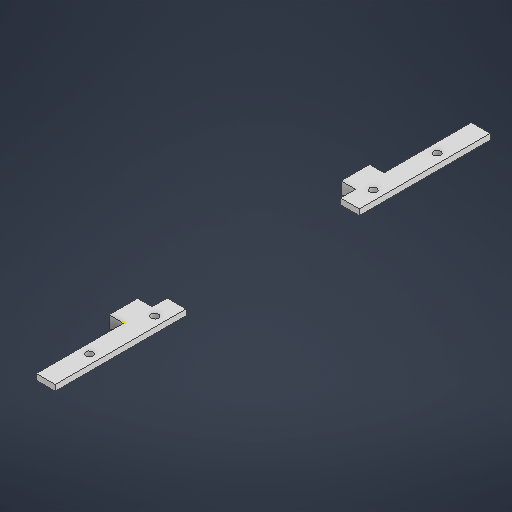
# Autodesk Inventor part: mocowanie do pługu
Saved by Autodesk Inventor 2026.2 (Build 302298010, 298A)
## iProperties
Created: 2026-05-09
Part Number: mocowanie do pługu
Material: Ogólny
Document SubType Name: Modeling
Designer: karol
Density: 1 g/cm^3
Appearance: Domyślna
Author: karol
Autodesk Inventor part; units mm, degrees
ref_plane "YZ Plane" through (0, 0, 0) normal (1, 0, 0) x (0, 1, 0)
ref_plane "XZ Plane" through (0, 0, 0) normal (0, 1, 0) x (-1, 0, 0)
ref_plane "XY Plane" through (0, 0, 0) normal (0, 0, 1) x (1, 0, 0)
sketch "Sketch21" plane through (0, 0, 0) normal (0, 1, 0) x (-1, 0, 0)
  line L0 (0, 0) -> (5, 0)
  line L1 (5, 0) -> (5, -9.8)
  line L2 (5, -9.8) -> (0, -9.8)
  line L3 (0, -9.8) -> (0, 0)
  line L4 (0, -79.8) -> (5, -79.8)
  line L5 (5, -79.8) -> (5, -89.6)
  line L6 (5, -89.6) -> (0, -89.6)
  line L7 (0, -89.6) -> (0, -79.8)
  dimension "d144" = 5
  dimension "d145" = 9.8
  dimension "d146" = 5
  dimension "d147" = 9.8
  dimension "d148" = 70
  constraints: 16 end point, 4 parallel, 2 horizontal, 2 perpendicular
  measures "d144" distance of L1.end L2.end
  measures "d145" distance of L0.end L1.end
  measures "d146" distance of L5.end L6.end
  measures "d147" distance of L4.end L5.end
  measures "d148" distance between parallel lines of L2 L4
extrude "Extrusion19" add sketch "Sketch21" along normal blind 4
sketch "Sketch22" plane through (0, 0, 0) normal (1, 0, 0) x (0, 0, -1)
  line L0 (9.8, 4) -> (0, 4) projected
  line L1 (9.8, 0) -> (9.8, 4) projected
  line L2 (0, 4) -> (9.8, 4)
  line L3 (9.8, 4) -> (9.8, 2)
  line L4 (9.8, 2) -> (0, 2)
  line L5 (0, 2) -> (0, 4)
  line L6 (9.8, 4) -> (15, 4)
  line L7 (15, 4) -> (15, 2)
  line L8 (15, 2) -> (9.8, 2)
  line L9 (9.8, 2) -> (9.8, 4)
  line L10 (0, 4) -> (-30, 4)
  line L11 (-30, 4) -> (-30, 2)
  line L12 (-30, 2) -> (0, 2)
  line L13 (0, 2) -> (0, 4)
  line L14 (89.6, 0) -> (89.6, 4) projected
  line L15 (79.8, 4) -> (89.6, 4)
  line L16 (89.6, 4) -> (89.6, 2)
  line L17 (89.6, 2) -> (79.8, 2)
  line L18 (79.8, 2) -> (79.8, 4)
  line L19 (79.8, 2) -> (74.6, 2)
  line L20 (74.6, 2) -> (74.6, 4)
  line L21 (74.6, 4) -> (79.8, 4)
  line L22 (79.8, 4) -> (79.8, 2)
  line L23 (89.6, 4) -> (119.6, 4)
  line L24 (119.6, 4) -> (119.6, 2)
  line L25 (119.6, 2) -> (89.6, 2)
  line L26 (89.6, 2) -> (89.6, 4)
  point P0 (0, 0)
  point P1 (9.8, 3)
  point P2 (0, 3)
  dimension "d151" = 9.8
  dimension "d152" = 5.2
  dimension "d153" = 30
  dimension "d154" = 5.2
  dimension "d155" = 30
  constraints: 48 end point, 12 parallel, 6 horizontal, 6 perpendicular, 4 midpoint, 2 point on line
  measures "d151" distance of point (9.8, 3) point (0, 3)
  measures "d152" distance of L7.end L8.end
  measures "d153" distance of L12.end L11.end
  measures "d154" distance of L20.end L21.end
  measures "d155" distance of L24.end L25.end
extrude "Extrusion20" add sketch "Sketch22" along normal blind 6.5
sketch "Sketch23" plane through (0, 4, 0) normal (0, 1, 0) x (1, 0, 0)
  point P0 (0, 0)
sketch "Sketch24" plane through (0, 4, 0) normal (0, 1, 0) x (1, 0, 0)
  circle A0 centre (3.25, -15) radius 1.25
  circle A1 centre (3.25, 7.5) radius 1.25
  line L0 (0, -30) -> (6.5, -30) projected
  line L1 (0, 0) -> (0, -30) projected
  line L2 (0, 15) -> (0, 9.8) projected
  circle A2 centre (3.25, 82.6) radius 1.25
  circle A3 centre (3.25, 104.6) radius 1.25
  line L3 (0, 119.6) -> (0, 89.6) projected
  line L4 (0, 119.6) -> (6.5, 119.6) projected
  point P0 (3.25, -30)
  point P1 (3.25, -30)
  point P2 (3.25, 119.6)
  point P3 (3.25, 119.6)
  dimension "d158" = 2.5
  dimension "d159" = 2.5
  dimension "d160" = 15
  dimension "d161" = 37.5
  dimension "d162" = 3.25
  dimension "d163" = 3.25
  dimension "d164" = 2.5
  dimension "d165" = 2.5
  dimension "d166" = 3.25
  dimension "d167" = 15
  dimension "d169" = 37
  dimension "d170" = 3.25
  constraints: 4 centre point, 4 midpoint
  measures "d158" diameter of A0
  measures "d159" diameter of A1
  measures "d160" distance of point (3.25, -30) A0.centre
  measures "d161" distance of point (3.25, -30) A1.centre
  measures "d162" distance from line of L1 A0.centre
  measures "d163" distance from line of L2 A1.centre
  measures "d164" diameter of A2
  measures "d165" diameter of A3
  measures "d166" distance from line of L3 A3.centre
  measures "d167" distance of point (3.25, 119.6) A3.centre
  measures "d169" distance of point (3.25, 119.6) A2.centre
  measures "d170" distance from line of L3 A2.centre
extrude "Extrusion21" cut sketch "Sketch24" against normal blind 2
body "Solid2"
